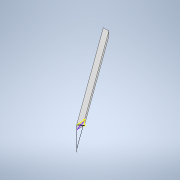
# Autodesk Inventor part: UpperExteriorDiagonal
Saved by Autodesk Inventor 2020.1 (Build 241239000, 239)
## iProperties
Created: 2020-02-04
Part Number: UpperExteriorDiagonal
Material: Generic
Document SubType Name: Modeling
Designer: super
Density: 1 g/cm^3
Appearance: Default
Author: super
Autodesk Inventor part; units mm, degrees
ref_plane "YZ Plane" through (0, 0, 0) normal (1, 0, 0) x (0, 1, 0)
ref_plane "XZ Plane" through (0, 0, 0) normal (0, 1, 0) x (-1, 0, 0)
ref_plane "XY Plane" through (0, 0, 0) normal (0, 0, 1) x (1, 0, 0)
sketch "Sketch1" plane through (0, 0, 0) normal (0, 1, 0) x (-1, 0, 0)
  line L0 (0, 0) -> (91.1067, -125.3976)
  line L1 (0, 0) -> (155, 0) construction
  line L2 (91.1067, -125.3976) -> (98.9557, -125.3976)
  line L3 (98.9557, -125.3976) -> (0, 10.8033)
  line L4 (0, 10.8033) -> (0, 0)
  dimension "d0" = 155
  dimension "d1" = 54
  constraints: 10 end point, 2 horizontal, 1 equal length, 1 perpendicular
  measures "d0" distance of L0.start L0.end
  measures "d1" angle of L0 L1
extrude "Extrusion1" add sketch "Sketch1" along normal blind 6.35
sketch "Sketch2" plane through (0, 6.35, 0) normal (0, 1, 0) x (1, 0, 0)
  point P0 (0, 0)
sketch "Sketch3" plane through (0, 0, 10.8033) normal (1, 0, 0) x (0, 0, -1)
  line L0 (0, 6.35) -> (10.8033, 6.35) projected
  line L1 (10.8033, 0) -> (10.8033, 6.35) projected
  line L2 (0, 6.35) -> (10.8033, 0)
  line L3 (10.8033, 6.35) -> (0, 0)
  constraints: 4 end point
sketch "Sketch4" plane through (0, 0, 10.8033) normal (1, 0, 0) x (0, 0, -1)
  point P0 (10.8033, 0)
sketch "Sketch5" plane through (0, 0, 10.8033) normal (1, 0, 0) x (0, 0, -1)
  point P0 (10.8033, 0)
body "Solid1"
